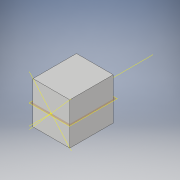
# Autodesk Inventor part: Solenoid
Saved by Autodesk Inventor 2017 (Build 210142000, 142)
## iProperties
Created: 2018-11-23
Part Number: Solenoid
Material: Generic
Document SubType Name: Modeling
Designer: Eric the Great
Density: 1 g/cm^3
Appearance: Default
Author: Eric the Great
Autodesk Inventor part; units mm, degrees
ref_plane "YZ Plane" through (0, 0, 0) normal (1, 0, 0) x (0, 1, 0)
ref_plane "XZ Plane" through (0, 0, 0) normal (0, 1, 0) x (-1, 0, 0)
ref_plane "XY Plane" through (0, 0, 0) normal (0, 0, 1) x (1, 0, 0)
sketch "Sketch2" plane through (0, 0, 0) normal (0, 1, 0) x (-1, 0, 0)
  line L0 (-9.4955, 22.0084) -> (12.5045, 22.0084)
  line L1 (12.5045, 22.0084) -> (12.5045, 48.0084)
  line L2 (12.5045, 48.0084) -> (-9.4955, 48.0084)
  line L3 (-9.4955, 48.0084) -> (-9.4955, 22.0084)
  point P0 (0, 0)
  dimension "d0" = 26
  dimension "d1" = 22
  constraints: 8 end point, 2 parallel, 1 horizontal, 1 perpendicular
  measures "d0" distance of L2.end L0.start
  measures "d1" distance of L1.end L2.end
extrude "Extrusion1" add sketch "Sketch2" along normal mid plane 25
ref_plane "Work Plane1" through (-1.5045, 0, 48.0084) normal (0, 1, 0) x (0, 0, 1)
sketch "Sketch5" plane through (9.4955, 12.5, 22.0084) normal (0, 0, -1) x (-1, 0, 0)
  point P0 (9.4955, -12.5)
body "Solid1"
